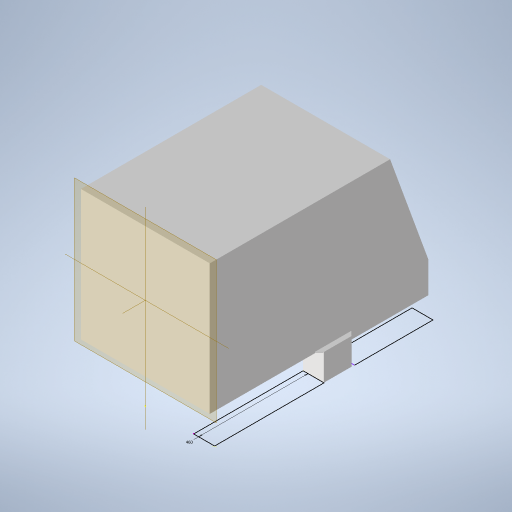
# Autodesk Inventor part: body_collisio
Saved by Autodesk Inventor 2023 (Build 270158000, 158)
## iProperties
Created: 2023-08-24
Part Number: body_collisio
Material: Generic
Document SubType Name: Modeling
Designer: chriboehm
Density: 1 g/cm^3
Appearance: Default
Author: chriboehm
Autodesk Inventor part; units mm, degrees
ref_plane "YZ Plane" through (0, 0, 0) normal (1, 0, 0) x (0, 1, 0)
ref_plane "XZ Plane" through (0, 0, 0) normal (0, 1, 0) x (-1, 0, 0)
ref_plane "XY Plane" through (0, 0, 0) normal (0, 0, 1) x (1, 0, 0)
ref_plane "Work Plane1" through (0, 0, 0) normal (0, 0, 1) x (1, 0, 0)
sketch "Sketch1" plane through (0, 0, 0) normal (0, 0, 1) x (1, 0, 0)
  line L0 (271, 270) -> (271, -270) projected
  line L1 (-271, 270) -> (271, 270) projected
  line L2 (271, -273) -> (271, -270) projected
  line L3 (262.1457, -273) -> (289.056, -273) projected
  line L4 (290.5196, -278) -> (290.5196, -273) projected
  arc A0 (221.5544, -380.4278) -> (259.4491, -380.4278) centre (240.5018, -345.2) ccw
  line L5 (-86.5386, -360.7555) -> (157.2553, -305.3974) projected
  line L6 (-260.1199, -400.1704) -> (-86.5386, -360.7555) projected
  line L7 (-265.6803, -388.102) -> (-276.918, -338.6119) projected
  line L8 (-271, -270) -> (-271, 270) projected
  line L9 (-278.1369, -338.8887) -> (-266.8992, -388.3788) projected
  line L10 (-260.1199, -400.1704) -> (-266.8992, -388.3788)
  line L11 (-266.8992, -388.3788) -> (-278.1369, -338.8887)
  line L12 (-278.1369, -338.8887) -> (-271, -273)
  line L13 (-271, -273) -> (-271, 270)
  line L14 (-271, 270) -> (271, 270)
  line L15 (271, 270) -> (271, -273)
  line L16 (271, -273) -> (290.5196, -273)
  line L17 (290.5196, -273) -> (290.5196, -303.7097)
  line L18 (290.5196, -303.7097) -> (290.5196, -384.6531)
  line L19 (205.5016, -303.2) -> (205.4838, -303.7097) projected
  line L20 (290.5196, -384.6531) -> (202.6414, -384.6531)
  line L21 (202.6414, -305.3974) -> (202.6414, -384.6531)
  line L22 (202.6414, -305.3974) -> (157.2553, -305.3974)
  line L23 (157.2553, -305.3974) -> (-260.1199, -400.1704)
  point P0 (0, 0)
  constraints: 26 end point, 4 collinear, 3 vertical, 2 point on circle, 1 centre point, 1 horizontal, 1 perpendicular, 1 point on line, 7 other
ref_plane "Work Plane2" through (-266.75, -268.75, -918) normal (0, 0, -1) x (0, 1, 0)
extrude "Extrusion1" add sketch "Sketch1" against normal up to surface (918 mm away) contours L0 L2 L3 L16 L4 L17 L18 L20 L21 L22 L5 L6 L10 L9 L12 L13 L8 L1
sketch "Sketch2" plane through (202.6414, -384.6531, 0) normal (-1, 0, 0) x (0, 0, 1)
  line L0 (0, 0) -> (0, 111.6531) projected
  line L1 (0, 79.2557) -> (-918, 79.2557) projected
  line L2 (0, 0) -> (-618, 0)
  line L3 (-618, 0) -> (-618, 79.2557)
  line L4 (-618, 79.2557) -> (0, 79.2557)
  line L5 (0, 79.2557) -> (0, 0)
  line L6 (-623, -15.5173) -> (-623, 23.8976) projected
  line L7 (-918, 79.2557) -> (-918, 0) projected
  line L8 (0, 79.2557) -> (0, 0) projected
  line L9 (0, 0) -> (-618, 0)
  line L10 (-618, 0) -> (-618, -151.7168)
  line L11 (-618, -151.7168) -> (0, -151.7168)
  line L12 (0, -151.7168) -> (0, 0)
  line L13 (0, 111.6531) -> (-918, 111.6531) projected
  line L14 (0, 79.2557) -> (-618, 79.2557)
  line L15 (-618, 79.2557) -> (-618, 106.6531)
  line L16 (-618, 106.6531) -> (0, 106.6531)
  line L17 (0, 106.6531) -> (0, 79.2557)
  point P0 (0, 384.6531)
  point P1 (-618, 0)
  point P2 (0, 106.6531)
  dimension "d2" = 300
  dimension "d5" = 300
  dimension "d18" = 5
  constraints: 24 end point, 6 parallel, 3 horizontal, 3 perpendicular, 1 point on line
  measures "d2" distance between parallel lines of L7 L3
  measures "d5" distance between parallel lines of L7 L10
  measures "d18" distance from line of L16 L0.end
extrude "Extrusion2" cut sketch "Sketch2" along normal through all
sketch "Sketch3" plane through (202.6414, -384.6531, 0) normal (0, -1, 0) x (1, 0, 0)
  line L0 (0, -618) -> (0, -918) projected
  line L1 (87.8782, 0) -> (0, 0)
  line L2 (0, 0) -> (0, -460)
  line L3 (0, -460) -> (87.8782, -460)
  line L4 (87.8782, -460) -> (87.8782, 0)
  line L5 (0, -918) -> (87.8782, -918) projected
  line L6 (0, 0) -> (0, -918) projected
  line L7 (87.8782, -918) -> (0, -918)
  line L8 (0, -918) -> (0, -588.5734)
  line L9 (0, -588.5734) -> (87.8782, -588.5734)
  line L10 (87.8782, -588.5734) -> (87.8782, -918)
  point P0 (-202.6414, 0)
  dimension "d8" = 460
  constraints: 16 end point, 4 parallel, 2 horizontal, 2 perpendicular, 2 point on line
  measures "d8" distance between parallel lines of L1 L3
extrude "Extrusion3" cut sketch "Sketch3" against normal up to surface (106.6531 mm away) contours L4 L3 L2 L1
sketch "Sketch4" plane through (271, -273, 0) normal (0, 1, 0) x (1, 0, 0)
  line L0 (19.5196, 0) -> (19.5196, 918) projected
  line L1 (-8.8543, 433.3976) -> (18.056, 460.3216) projected
  line L2 (0, 0) -> (0, 918) projected
  line L3 (19.5196, 0) -> (0, 0) projected
  line L4 (18.056, 577.2146) -> (-8.8543, 604.1385) projected
  line L5 (19.5196, 918) -> (0, 918) projected
  line L6 (19.5196, 918) -> (19.5196, 577.2146)
  line L7 (19.5196, 460) -> (19.5196, 918) projected
  line L8 (18.056, 577.2146) -> (19.5196, 577.2146)
  line L9 (18.056, 577.2146) -> (0, 595.2798)
  line L10 (0, 0) -> (0, 918) projected
  line L11 (0, 595.2798) -> (0, 918)
  line L12 (0, 918) -> (19.5196, 918)
  line L13 (18.056, 460.3216) -> (19.5196, 460.3216)
  line L14 (19.5196, 460.3216) -> (19.5196, 0)
  line L15 (19.5196, 0) -> (0, 0)
  line L16 (0, 0) -> (0, 442.2564)
  line L17 (0, 442.2564) -> (18.056, 460.3216)
  point P0 (-271, 0)
  point P1 (19.5196, 588.5734)
  point P2 (19.5196, 577.2146)
  point P3 (0, 595.2798)
  constraints: 20 end point, 6 point on line, 3 collinear, 3 perpendicular
extrude "Extrusion4" cut sketch "Sketch4" against normal up to surface (111.6531 mm away) contours L3 L2 L1 L13 L0 | L8 L4 L2 L5 L0
sketch "Sketch5" plane through (-260.1199, -400.1704, -918) normal (0.2214323, -0.9751758, 0) x (0.9751758, 0.2214323, 0)
  line L0 (-4, 291) -> (428, 291)
  line L1 (428, 291) -> (428, 14)
  line L2 (428, 14) -> (-4, 14)
  line L3 (-4, 14) -> (-4, 291)
  line L4 (0, 292) -> (178, 292) projected
  line L5 (250, 13) -> (0, 13) projected
  line L6 (-4, 300) -> (-4, 0) projected
  line L7 (428, 300) -> (428, 0) projected
  point P0 (342.2733, 918)
  dimension "d11" = 1
  dimension "d12" = 1
  constraints: 8 end point, 2 collinear, 2 parallel, 1 horizontal, 1 perpendicular
  measures "d11" distance between parallel lines of L4 L0
  measures "d12" distance between parallel lines of L5 L2
extrude "Extrusion5" cut sketch "Sketch5" against normal blind 9
sketch "Sketch6" plane through (-274.5092, -305.3974, 0) normal (0, -1, 0) x (1, 0, 0)
  line L0 (14.3893, -627) -> (431.7645, -627) projected
  line L1 (423.6845, -627) -> (501.5092, -627)
  line L2 (501.5092, -627) -> (501.5092, -904)
  line L3 (501.5092, -904) -> (423.6845, -904)
  line L4 (423.6845, -904) -> (423.6845, -627)
  line L5 (502.5092, -657) -> (502.5092, -620) projected
  line L6 (502.5092, -911) -> (502.5092, -874) projected
  point P0 (274.5092, 0)
  dimension "d15" = 1
  constraints: 8 end point, 2 parallel, 1 horizontal, 1 perpendicular, 1 point on line
  measures "d15" distance between parallel lines of L5 L2
extrude "Extrusion6" cut sketch "Sketch6" against normal blind 9
extrude "Extrusion7" cut sketch "Sketch3" against normal up to surface (79.2557 mm away) contours L6 L9 L10 L5 L0
sketch "Sketch7" plane through (-271, -273, 0) normal (-1, 0, 0) x (0, 0, 1)
  line L0 (-918, 543) -> (-918, 0) projected
  line L1 (-918, 100) -> (-758, 543)
  line L2 (0, 543) -> (-918, 543) projected
  line L3 (-918, 543) -> (-758, 543)
  line L4 (-918, 543) -> (-918, 100)
  point P0 (0, 273)
  dimension "d21" = 100
  dimension "d22" = 160
  constraints: 6 end point, 2 point on line, 1 horizontal, 1 perpendicular
  measures "d21" distance of L1.start L0.end
  measures "d22" distance from line of L0 L1.end
extrude "Extrusion8" cut sketch "Sketch7" against normal through all
equation "\"d5\" = d2"
equation "\"d12\" = d11"
body "Solid1"
